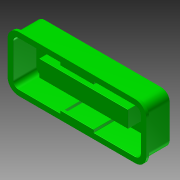
# Autodesk Inventor part: T9 One Block Socket
Saved by Autodesk Inventor 2015 (Build 190159000, 159)
## iProperties
Created: 2012-02-21
Part Number: T9 One Block Socket
Material: Generic
Document SubType Name: Modeling
Designer: Thom Tremblay
Density: 1 g/cm^3
Appearance: Dark Green
Author: Thom Tremblay
Autodesk Inventor part; units mm, degrees
sketch "Sketch1" plane through (0, 0, 0) normal (0, 0, 1) x (1, 0, 0)
  line L0 (0, 0) -> (31.75, 0)
  line L1 (31.75, 0) -> (31.75, 12.7)
  line L2 (31.75, 12.7) -> (0, 12.7)
  line L3 (0, 12.7) -> (0, 0)
  dimension "d0" = 31.75
  dimension "d1" = 12.7
  constraints: 8 end point, 2 parallel, 1 horizontal, 1 perpendicular
  measures "d0" distance of L2.end L1.end
  measures "d1" distance of L1.end L0.end
extrude "Extrusion1" add sketch "Sketch1" along normal blind 11.938
fillet "Fillet1" radius 5.08 1 edges at (31.75, 12.7, 5.969)
shell "Shell1" thickness 2.54 removed faces 3 at (0, 8.4667, 3.9793) at (19.4733, 4.2333, 11.938) at (10.5833, 0, 7.9587) ; own thickness 1.27 on faces at (19.4733, 4.2333, 0)
sketch "Sketch2" plane through (0, 0, 1.27) normal (0, 0, 1) x (1, 0, 0)
  line L0 (29.21, 0) -> (0, 0) construction
  line L1 (11.303, 0) -> (22.987, 0)
  line L2 (22.987, 0) -> (22.987, 5.7977)
  line L3 (22.987, 5.7977) -> (11.303, 5.7977)
  line L4 (11.303, 5.7977) -> (11.303, 0)
  dimension "d7" = 11.684
  dimension "d8" = 5.7977
  dimension "d26" = 11.303
  constraints: 8 end point, 2 parallel, 1 horizontal, 1 perpendicular, 1 point on line
  measures "d7" distance of L1.start L1.end
  measures "d8" distance of L1.end L2.end
  measures "d26" distance from line of L0.end L4
ref_plane "Work Plane1" through (0, 0, 11.0998) normal (0, 0, 1) x (1, 0, 0)
shell "Shell2" thickness 1.27 removed faces 6 at (17.78, 12.7, 3.9793) at (28.5259, 12.3488, 3.9793) at (31.75, 2.54, 7.9587) at (19.4733, 4.2333, 0) at (0, 11.8533, 4.4027) at (20.32, 0, 0.4233)
sketch "Sketch4" plane through (0, 10.16, 11.938) normal (0, -1, 0) x (1, 0, 0)
  line L0 (0, -10.668) -> (0, 0) projected
  line L1 (0, 0) -> (7.62, 0)
  line L2 (7.62, 0) -> (7.62, -10.668)
  line L3 (7.62, -10.668) -> (0, -10.668)
  line L4 (0, -10.668) -> (0, 0)
  point P0 (0, -11.938)
  dimension "d29" = 7.62
  constraints: 8 end point, 2 parallel, 1 horizontal, 1 perpendicular
  measures "d29" distance of L0.end L1.end
extrude "Extrusion5" add sketch "Sketch4" along normal blind 1.27
ref_plane "Work Plane3" through (0, 0, 10.668) normal (0, 0, 1) x (1, 0, 0)
sketch "Sketch5" plane through (0, 0, 10.668) normal (0, 0, 1) x (1, 0, 0)
  line L0 (0, 8.89) -> (6.858, 8.89)
  line L1 (6.858, 8.89) -> (6.858, 10.16)
  line L2 (6.858, 10.16) -> (0, 10.16)
  line L3 (0, 10.16) -> (0, 8.89)
  line L4 (7.62, 10.16) -> (7.62, 8.89) projected
  point P0 (0, 0)
  dimension "d33" = 1.27
  dimension "d34" = 0.762
  constraints: 8 end point, 2 parallel, 1 horizontal, 1 perpendicular
  measures "d33" distance of L2.end L0.start
  measures "d34" distance between parallel lines of L4 L1
extrude "Extrusion6" cut sketch "Sketch5" against normal through all
ref_plane "Work Plane4" through (0, 0, 8.89) normal (0, 0, 1) x (1, 0, 0)
sketch "Sketch6" plane through (0, 0, 1.27) normal (0, 0, 1) x (1, 0, 0)
  line L0 (0, 0) -> (20.32, 0)
  line L1 (20.32, 0) -> (20.32, 3.81)
  line L2 (20.32, 3.81) -> (0, 3.81)
  line L3 (0, 3.81) -> (0, 0)
  dimension "d38" = 20.32
  dimension "d39" = 3.81
  constraints: 8 end point, 2 parallel, 1 horizontal, 1 perpendicular
  measures "d38" distance of L2.end L1.end
  measures "d39" distance of L0.end L1.end
extrude "Extrusion7" add sketch "Sketch6" along normal up to surface (7.62 mm away)
fillet "Fillet8" radius 0.127 10 edges at (20.32, 1.905, 8.89) (10.16, 3.81, 8.89) (20.32, 3.81, 5.08) (28.4661, 9.4161, 11.938) (17.145, 10.16, 11.938) (29.21, 3.81, 11.938) (7.62, 9.525, 11.938) (3.81, 8.89, 11.938) (7.62, 8.89, 6.604) (7.62, 10.16, 6.604)
mirror "Mirror3" about plane through (0, 0, 0) normal (-1, 0, 0)
mirror "Mirror4" about plane through (31.75, 0, 0) normal (0, -1, 0)
body "Solid1"
